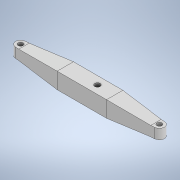
# Autodesk Inventor part: parallel_bar_long_no_hole_v1
Saved by Autodesk Inventor 2022 (Build 260153000, 153)
## iProperties
Created: 2022-05-22
Part Number: parallel_bar_long_no_hole_v1
Material: Generic
Document SubType Name: Modeling
Designer: kylem
Density: 1 g/cm^3
Appearance: Default
Author: kylem
Autodesk Inventor part; units mm, degrees
ref_plane "YZ Plane" through (0, 0, 0) normal (1, 0, 0) x (0, 1, 0)
ref_plane "XZ Plane" through (0, 0, 0) normal (0, 1, 0) x (-1, 0, 0)
ref_plane "XY Plane" through (0, 0, 0) normal (0, 0, 1) x (1, 0, 0)
sketch "Sketch1" plane through (0, 0, 0) normal (0, 1, 0) x (-1, 0, 0)
  line L0 (0, 0) -> (60, 0)
  line L1 (60, 0) -> (60, -4)
  line L2 (60, -4) -> (0, -4)
  line L3 (0, -4) -> (0, 0)
  dimension "d0" = 60
  dimension "d1" = 4
  constraints: 8 end point, 2 parallel, 1 horizontal, 1 perpendicular
  measures "d0" distance of L1.end L2.end
  measures "d1" distance of L0.end L1.end
extrude "Extrusion1" add sketch "Sketch1" along normal blind 4
sketch "Sketch2" plane through (0, 4, 0) normal (0, 1, 0) x (1, 0, 0)
  line L0 (0, 0) -> (0, 4) projected
  line L1 (0, 2) -> (-2, 2)
  circle A0 centre (-2, 2) radius 1
  line L2 (0, 4) -> (-60, 4) projected
  line L3 (-30, 4) -> (-30, 1.3223)
  circle A1 centre (-58, 2) radius 1
  dimension "d4" = 2
  dimension "d5" = 2
  constraints: 4 end point, 2 centre point, 2 midpoint, 1 coincident, 1 horizontal, 1 symmetric about line, 1 vertical, 1 other
  measures "d4" distance of L1.start L1.end
  measures "d5" diameter of A0
extrude "Extrusion2" cut sketch "Sketch2" against normal blind 4
sketch "Sketch4" plane through (0, 4, 0) normal (0, 1, 0) x (1, 0, 0)
  circle A0 centre (-2, 2) radius 1 projected
  circle A1 centre (-2, 2) radius 2
  line L0 (0, 4) -> (-60, 4) projected
  line L1 (-60, 0) -> (0, 0) projected
  line L2 (-2, 4) -> (0, 4)
  line L3 (0, 4) -> (0, 0)
  line L4 (0, 0) -> (-2, 0)
  line L5 (-2, 0) -> (-2, 4)
  line L6 (-60, 4) -> (0, 4)
  line L7 (-30, 4) -> (-30, 6.9256)
  circle A2 centre (-58, 2) radius 1
  circle A3 centre (-58, 2) radius 2
  line L8 (-60, 4) -> (0, 4)
  line L9 (0, 0) -> (-60, 0)
  line L10 (-58, 4) -> (-60, 4)
  line L11 (-60, 4) -> (-60, 0)
  line L12 (-60, 0) -> (-58, 0)
  line L13 (-58, 0) -> (-58, 4)
  line L14 (0, 4) -> (-60, 4)
  point P0 (0, 2)
  point P1 (-60, 2)
  constraints: 26 end point, 9 symmetric about line, 2 coincident, 2 parallel, 2 point on line, 2 vertical, 1 centre point, 1 collinear, 1 horizontal, 1 midpoint, 1 perpendicular, 7 other
extrude "Extrusion5" cut sketch "Sketch4" against normal blind 10 contours L0 L3 A1 | A1 L3 L1 | L1 L11 A3 | A3 L11 L0
sketch "Sketch6" plane through (0, 4, 0) normal (0, 1, 0) x (1, 0, 0)
  line L0 (-2, 4) -> (-58, 4) projected
  line L1 (-30, 4) -> (-30, 6)
  line L2 (-30, 6) -> (-58.1421, 3.9949)
  arc A0 (-58, 4) -> (-58, 0) centre (-58, 2) ccw projected
  circle A1 centre (-58, 2) radius 1 projected
  line L3 (-58, 2) -> (-47.7082, 2)
  line L4 (-30, 6) -> (-1.8579, 3.9949)
  line L5 (-30, -2) -> (-58.1421, 0.0051)
  line L6 (-30, -2) -> (-1.8579, 0.0051)
  line L7 (-58.1421, 0.0051) -> (-1.8579, 0.0051)
  line L8 (-1.8579, 3.9949) -> (-58.1421, 3.9949)
  point P0 (0, 0)
  dimension "d27" = 2
  constraints: 16 end point, 4 symmetric about line, 2 horizontal, 1 midpoint, 1 parallel, 1 point on circle, 1 tangent, 1 vertical
  measures "d27" distance of L1.start L1.end
extrude "Extrusion7" add sketch "Sketch6" against normal blind 4 contours L1 L4 L8 A0 L0 | L0 A0 L2 L1 | L5 L7 L6
chamfer "Chamfer1" distance 10 angle 45 2 edges at (-30, 2, -6) (-30, 2, 2)
ref_plane "Work Plane1" through (-20.0253, 0, -2) normal (0, 0, -1) x (-1, 0, 0)
sketch "Sketch7" plane through (-20.0253, 0, -2) normal (0, 0, -1) x (-1, 0, 0)
  line L0 (-18.1674, 4) -> (-18.1674, 0) projected
  line L1 (-18.1674, 4) -> (-16.6674, 4)
  line L2 (-18.1674, 4) -> (0, 4) projected
  line L3 (38.1168, 4) -> (38.1168, 0) projected
  line L4 (38.1168, 0) -> (38.1168, 4)
  line L5 (38.1168, 2) -> (33.6087, 2)
  line L6 (38.1168, 0) -> (-18.1674, 0)
  line L7 (-17.0253, 0) -> (-19.0253, 0) projected
  line L8 (19.9494, 0) -> (0, 0) projected
  line L9 (9.9747, 0) -> (9.9747, -6.0708)
  line L10 (9.9747, 0) -> (9.9747, 4)
  line L11 (0, 4) -> (19.9494, 4) projected
  line L12 (9.9747, 4) -> (9.9747, 6)
  line L13 (19.9494, 4) -> (38.1168, 4) projected
  line L14 (9.9747, 6) -> (-16.6674, 4)
  line L15 (9.9747, 6) -> (36.6168, 4)
  line L16 (9.9747, -2) -> (-16.6674, 0)
  line L17 (9.9747, -2) -> (36.6168, 0)
  line L18 (36.6168, 4) -> (-16.6674, 4)
  line L19 (-16.6674, 4) -> (-16.6674, 0)
  line L20 (-16.6674, 0) -> (36.6168, 0)
  line L21 (36.6168, 0) -> (36.6168, 4)
  line L22 (36.6168, 4) -> (-16.6674, 4)
  line L23 (-16.6674, 0) -> (36.6168, 0)
  line L24 (19.9494, 0) -> (38.1168, 0) projected
  point P0 (-20.0253, 0)
  point P1 (-16.6674, 0)
  point P2 (36.6168, 0)
  point P3 (36.6168, 4)
  dimension "d33" = 1.5
  dimension "d34" = 2
  constraints: 34 end point, 4 collinear, 4 symmetric about line, 3 midpoint, 2 horizontal, 2 parallel, 2 point on line, 1 perpendicular, 1 vertical
  measures "d33" distance of L0.start L1.end
  measures "d34" distance of L10.end L12.end
extrude "Extrusion8" add sketch "Sketch7" along normal mid plane 10 contours L14 L12 L11 L2 | L15 L13 L11 L12 | L6 L9 L16 | L9 L6 L17
sketch "Sketch8" plane through (-1.8579, 0, -3.9949) normal (0.0710674, 0, -0.9974715) x (-0.9974715, 0, -0.0710674)
  line L0 (35.9891, -12.6752) -> (-6.3652, -12.6752)
  line L1 (-6.3652, -12.6752) -> (-6.3652, 25.3058)
  line L2 (-6.3652, 25.3058) -> (35.9891, 25.3058)
  line L3 (35.9891, 25.3058) -> (35.9891, -12.6752)
  point P0 (-2.1371, 0)
  constraints: 8 end point, 2 parallel, 1 horizontal, 1 perpendicular
extrude "Extrusion9" cut sketch "Sketch8" along normal blind 10
sketch "Sketch9" plane through (-58.1421, 0, -3.9949) normal (-0.0710674, 0, -0.9974715) x (-0.9974715, 0, 0.0710674)
  line L0 (14.3084, 30.8799) -> (-35.9068, 30.8799)
  line L1 (-35.9068, 30.8799) -> (-35.9068, -25.4425)
  line L2 (-35.9068, -25.4425) -> (14.3084, -25.4425)
  line L3 (14.3084, -25.4425) -> (14.3084, 30.8799)
  point P0 (-57.7112, 0)
  constraints: 8 end point, 2 parallel, 1 horizontal, 1 perpendicular
extrude "Extrusion10" cut sketch "Sketch9" along normal blind 10
sketch "Sketch10" plane through (-20.0253, 0, -5.2893) normal (0, 0, -1) x (-1, 0, 0)
  line L0 (23.8295, 22.9885) -> (-8.7859, 22.9885)
  line L1 (-8.7859, 22.9885) -> (-8.7859, -15.4672)
  line L2 (-8.7859, -15.4672) -> (23.8295, -15.4672)
  line L3 (23.8295, -15.4672) -> (23.8295, 22.9885)
  point P0 (-20.0253, 0)
  constraints: 8 end point, 2 parallel, 1 horizontal, 1 perpendicular
extrude "Extrusion11" cut sketch "Sketch10" along normal blind 10
ref_plane "Work Plane2" through (-39.9747, -1.2512, -2) normal (0, 0, -1) x (-1, 0, 0)
mirror "Mirror1" about plane through (-39.9747, -1.2512, -2) normal (0, 0, -1) of "Extrusion9", "Extrusion10", "Extrusion11"
chamfer "Chamfer2" distance 10 angle 45 2 edges at (-30, 6, -2) (-30, -2, -2)
sketch "Sketch11" plane through (-39.9719, 5.2514, 1.2893) normal (0, 1, 0) x (1, 0, 0)
  circle A0 centre (37.9719, 3.2893) radius 1 projected
  line L0 (37.9719, 3.2893) -> (12.9719, 3.2893)
  circle A1 centre (12.9719, 3.2893) radius 1.1
  point P0 (39.9719, 1.2893)
  dimension "d46" = 25
  dimension "d47" = 2.2
  constraints: 2 end point, 1 centre point, 1 coincident, 1 horizontal
  measures "d46" distance of L0.start L0.end
  measures "d47" diameter of A1
extrude "Extrusion12" cut sketch "Sketch11" against normal blind 10 contours A1
body "Solid1"
